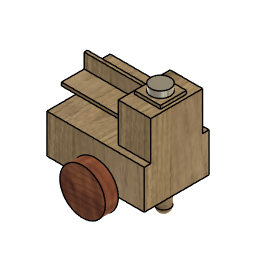
final_1100427 v4 (Autodesk Fusion 360 design; units mm, degrees)
Autodesk Fusion 360 part; units mm, degrees
sketch "Sketch1" plane through (0, 0, 0) normal (0, 0, 1) x (1, 0, 0)
  line L0 (75, 50) -> (-75, 50)
  line L1 (-75, 50) -> (-75, -50)
  line L2 (-75, -50) -> (75, -50)
  line L3 (75, -50) -> (75, 50)
  line L4 (75, 50) -> (-75, -50) construction
  line L5 (-75, 50) -> (75, -50) construction
  constraint horizontal L0
  constraint perpendicular L0 L1
  constraint parallel L0 L2
  constraint parallel L1 L3
  constraint coincident L4 origin
  constraint coincident L5 origin
extrude "Extrude1" add sketch "Sketch1" along normal blind 60 makes body 1
sketch "Sketch2" plane through (0, -50, 0) normal (0, -1, 0) x (1, 0, 0)
  line L0 (-75, 0) -> (75, 0)
  line L1 (75, 0) -> (75, 60)
  line L2 (75, 60) -> (-75, 60)
  line L3 (-75, 60) -> (-75, 0)
  circle A0 centre (0, 0) radius 35
  dimension "d3" = 70
  constraint coincident A0.centre origin
  measures "d3" diameter of A0
extrude "Extrude2" add sketch "Sketch2" along normal blind 20 separate body contours L0 A0 | L0 A0 makes body 2
sketch "Sketch3" plane through (0, 50, 0) normal (0, 1, 0) x (-1, 0, 0)
  line L0 (-75, 0) -> (75, 0)
  line L1 (75, 0) -> (75, 60)
  line L2 (75, 60) -> (-75, 60)
  line L3 (-75, 60) -> (-75, 0)
  circle A0 centre (0, 0) radius 35
  dimension "d6" = 70
  constraint coincident A0.centre origin
  measures "d6" diameter of A0
extrude "Extrude3" add sketch "Sketch3" along normal blind 20 separate body contours L0 A0 | L0 A0 makes body 3
sketch "Sketch4" plane through (0, 0, 0) normal (0, 0, -1) x (1, 0, 0)
  line L0 (75, -50) -> (75, 50)
  line L1 (75, 50) -> (-75, 50)
  line L2 (-75, 50) -> (-75, -50)
  line L3 (-75, -50) -> (75, -50)
  circle A0 centre (55, 0) radius 10
  dimension "d9" = 20
  measures "d9" diameter of A0
sketch "Sketch5" plane through (0, 0, 0) normal (0, 0, -1) x (1, 0, 0)
  circle A0 centre (-55, 0) radius 10
  dimension "d10" = 20
  measures "d10" diameter of A0
extrude "Extrude4" add sketch "Sketch4" along normal blind 35 contours A0 bodies 1
extrude "Extrude5" add sketch "Sketch5" along normal blind 35 bodies 1
fillet "Fillet1" radius 10 1 faces at (52.2459, -1.8777, -35) on bodies 1
fillet "Fillet2" radius 10 1 faces at (-57.4613, -0.9283, -35) on bodies 1
move_body "Move1" bodies 1 2 3 to x (1, 0, 0) y (0, 1, 0) z (0, 0, 1) at (0, 0, 35)
sketch "Sketch6" plane through (0, 0, 95) normal (0, 0, 1) x (-1, 0, 0)
  line L0 (-75, 50) -> (-75, -50)
  line L1 (-75, -50) -> (75, -50)
  line L2 (75, -50) -> (75, 50)
  line L3 (75, 50) -> (-75, 50)
  line L4 (-25, -40) -> (-75, -40)
  line L5 (-75, -40) -> (-75, 40)
  line L6 (-75, 40) -> (-25, 40)
  line L7 (-25, 40) -> (-25, -40)
  line L8 (-25, -40) -> (-75, 40) construction
  line L9 (-75, -40) -> (-25, 40) construction
  point P0 (-50, 0)
  constraint horizontal L4
  constraint perpendicular L4 L5
  constraint parallel L4 L6
  constraint parallel L5 L7
  constraint coincident L8 P0
  constraint coincident L9 P0
extrude "Extrude6" add sketch "Sketch6" along normal blind 60 contours L0 L4 L5 L6 L7 bodies 1
shell "Shell1" thickness 10 removed faces 1 at (-75, 16.6667, 55) on bodies 1
sketch "Sketch7" plane through (0, 0, 95) normal (0, 0, 1) x (-1, 0, 0)
  line L0 (-25, -40) -> (-75, -40)
  line L1 (-75, -40) -> (-75, -50)
  line L2 (-75, -50) -> (75, -50)
  line L3 (75, -50) -> (75, 50)
  line L4 (75, 50) -> (-75, 50)
  line L5 (-75, 50) -> (-75, 40)
  line L6 (-75, 40) -> (-25, 40)
  line L7 (-25, 40) -> (-25, -40)
  line L8 (65, 2.5) -> (-25, 2.5)
  line L9 (-25, 2.5) -> (-25, -2.5)
  line L10 (-25, -2.5) -> (65, -2.5)
  line L11 (65, -2.5) -> (65, 2.5)
  line L12 (65, 2.5) -> (-25, -2.5) construction
  line L13 (-25, 2.5) -> (65, -2.5) construction
  point P0 (20, 0)
  dimension "d22" = 90
  dimension "d23" = 5
  constraint horizontal L8
  constraint perpendicular L8 L9
  constraint parallel L8 L10
  constraint parallel L9 L11
  constraint coincident L12 P0
  constraint coincident L13 P0
  measures "d22" distance of L9.end L10.end
  measures "d23" distance of L8.end L9.end
extrude "Extrude7" add sketch "Sketch7" along normal blind 60 contours L7 L8 L9 L10 L11 bodies 1
sketch "Sketch8" plane through (0, -2.5, 0) normal (0, -1, 0) x (1, 0, 0)
  line L0 (-65, 95) -> (25, 95)
  line L1 (25, 95) -> (25, 155)
  line L2 (25, 155) -> (-65, 155)
  line L3 (-65, 155) -> (-65, 95)
  line L4 (25, 132.5) -> (-65, 132.5)
  line L5 (-65, 132.5) -> (-65, 127.5)
  line L6 (-65, 127.5) -> (25, 127.5)
  line L7 (25, 127.5) -> (25, 132.5)
  line L8 (25, 132.5) -> (-65, 127.5) construction
  line L9 (-65, 132.5) -> (25, 127.5) construction
  point P0 (-20, 130)
  dimension "d26" = 90
  dimension "d27" = 5
  constraint horizontal L4
  constraint perpendicular L4 L5
  constraint parallel L4 L6
  constraint parallel L5 L7
  constraint coincident L8 P0
  constraint coincident L9 P0
  measures "d26" distance of L5.end L6.end
  measures "d27" distance of L4.end L5.end
extrude "Extrude8" add sketch "Sketch8" along normal blind 35 contours L1 L3 L4 L5 L6 L7 bodies 1
sketch "Sketch9" plane through (0, 2.5, 0) normal (0, 1, 0) x (-1, 0, 0)
  line L0 (-25, 95) -> (65, 95)
  line L1 (65, 95) -> (65, 155)
  line L2 (65, 155) -> (-25, 155)
  line L3 (-25, 155) -> (-25, 95)
  line L4 (65, 132.5) -> (-25, 132.5)
  line L5 (-25, 132.5) -> (-25, 127.5)
  line L6 (-25, 127.5) -> (65, 127.5)
  line L7 (65, 127.5) -> (65, 132.5)
  line L8 (65, 132.5) -> (-25, 127.5) construction
  line L9 (-25, 132.5) -> (65, 127.5) construction
  point P0 (20, 130)
  dimension "d30" = 90
  dimension "d31" = 5
  constraint horizontal L4
  constraint perpendicular L4 L5
  constraint parallel L4 L6
  constraint parallel L5 L7
  constraint coincident L8 P0
  constraint coincident L9 P0
  measures "d30" distance of L5.end L6.end
  measures "d31" distance of L4.end L5.end
extrude "Extrude9" add sketch "Sketch9" along normal blind 35 contours L1 L3 L4 L5 L6 L7 bodies 1
sketch "Sketch10" plane through (0, 0, 155) normal (0, 0, 1) x (-1, 0, 0)
  line L0 (-25, 40) -> (-75, 40)
  line L1 (-75, 40) -> (-75, -40)
  line L2 (-75, -40) -> (-25, -40)
  line L3 (-25, -40) -> (-25, -2.5)
  line L4 (-25, -2.5) -> (65, -2.5)
  line L5 (65, -2.5) -> (65, 2.5)
  line L6 (65, 2.5) -> (-25, 2.5)
  line L7 (-25, 2.5) -> (-25, 40)
  circle A0 centre (-50, 0) radius 20
  dimension "d34" = 40
  measures "d34" diameter of A0
sketch "Sketch11" plane through (0, 0, 155) normal (0, 0, 1) x (-1, 0, 0)
  line L0 (-25, 40) -> (-75, 40)
  line L1 (-75, 40) -> (-75, -40)
  line L2 (-75, -40) -> (-25, -40)
  line L3 (-25, -40) -> (-25, -2.5)
  line L4 (-25, -2.5) -> (65, -2.5)
  line L5 (65, -2.5) -> (65, 2.5)
  line L6 (65, 2.5) -> (-25, 2.5)
  line L7 (-25, 2.5) -> (-25, 40)
  line L8 (-30, 20) -> (-70, 20)
  line L9 (-70, 20) -> (-70, -20)
  line L10 (-70, -20) -> (-30, -20)
  line L11 (-30, -20) -> (-30, 20)
  line L12 (-30, 20) -> (-70, -20) construction
  line L13 (-70, 20) -> (-30, -20) construction
  point P0 (-50, 0)
  constraint horizontal L8
  constraint perpendicular L8 L9
  constraint parallel L8 L10
  constraint parallel L9 L11
  constraint coincident L12 P0
  constraint coincident L13 P0
extrude "Extrude11" add sketch "Sketch11" along normal blind 5 contours L8 L9 L10 L11 bodies 1
sketch "Sketch12" plane through (0, 0, 160) normal (0, 0, 1) x (-1, 0, 0)
  line L0 (-30, -20) -> (-30, 20)
  line L1 (-30, 20) -> (-70, 20)
  line L2 (-70, 20) -> (-70, -20)
  line L3 (-70, -20) -> (-30, -20)
  circle A0 centre (-50, 0) radius 15
  dimension "d39" = 30
  measures "d39" diameter of A0
extrude "Extrude12" add sketch "Sketch12" along normal blind 10 separate body contours A0 makes body 4
copy_body "Body->Comp1" bodies 1 removing the originals makes body 5 in component "base_link"
copy_body "Body->Comp2" bodies 2 removing the originals makes body 6 in component "right_wheel"
copy_body "Body->Comp3" bodies 3 removing the originals makes body 7 in component "left_wheel"
copy_body "Body->Comp4" bodies 4 removing the originals makes body 8 in component "lidar"
component "base_link" placed x (1, 0, 0) y (0, 1, 0) z (0, 0, 1) at (0, 0, 0)
component "right_wheel" placed x (0, 0, -1) y (0, 1, 0) z (1, 0, 0) at (-35, 0, 35)
component "left_wheel" placed x (1, 0, 0) y (0, 1, 0) z (0, 0, 1) at (0, 0, 0)
component "lidar" placed x (1, 0, 0) y (0, 1, 0) z (0, 0, 1) at (0, 0, 0)
named bodies: "base_link", "right_wheel", "left_wheel", "lidar"
